Autodesk Inventor part; units mm, degrees
(part 8 of 8)
  line L3438 (-10.9335, 45.6499) -> (-10.7357, 45.6499) construction
  line L3439 (-10.7357, 45.6499) -> (-10.6212, 45.7817) construction
  spline S1087 degree 2 poles (-10.6212, 45.7817) (-10.5171, 45.8997) (-10.5171, 46.0697) knots 0 0 0 1 1 1
  line L3440 (-10.6212, 45.7817) -> (-10.5171, 45.8997) construction
  line L3441 (-10.5171, 45.8997) -> (-10.5171, 46.0697) construction
  spline S1088 degree 2 poles (-10.5171, 46.0697) (-10.5171, 46.4409) (-10.878, 46.4791) knots 0 0 0 1 1 1
  line L3442 (-10.5171, 46.0697) -> (-10.5171, 46.4409) construction
  line L3443 (-10.5171, 46.4409) -> (-10.878, 46.4791) construction
  line L3444 (-10.878, 46.4791) -> (-11.1382, 46.4791)
  circle A70 centre (18.7074, -0.5093) radius 2.3333
  circle A71 centre (12.3767, 19.6182) radius 2.3333
  circle A72 centre (-8.6685, 63.1738) radius 2.3333
  circle A73 centre (7.9982, 63.1738) radius 2.3333
  circle A74 centre (3.1182, 73.7406) radius 2.3333
  circle A75 centre (-12.2369, -33.319) radius 2.3333
  circle A76 centre (17.5807, -32.3391) radius 2.3333
  circle A77 centre (0.1742, -74.3888) radius 1.8001
  circle A78 centre (7.1838, -70.3418) radius 1.8001
  circle A79 centre (-6.8355, -78.4359) radius 1.8
  circle A80 centre (-4.5413, -27.5841) radius 2.3333
  circle A81 centre (11.7025, 73.7406) radius 2.3333
  circle A82 centre (7.9982, 57.3405) radius 2.3333
  circle A83 centre (-8.6685, 57.3405) radius 2.3333
  circle A84 centre (18.7074, -8.8426) radius 2.3333
  circle A85 centre (-3.7926, -8.8426) radius 2.3333
  circle A86 centre (5.7517, 15.6786) radius 2.3333
  circle A87 centre (-17.0018, 57.3405) radius 2.3333
  circle A88 centre (-0.3351, 57.3405) radius 2.3333
  circle A89 centre (17.9982, 57.3405) radius 2.3333
  circle A90 centre (-12.2369, -27.5841) radius 2.3333
  circle A91 centre (17.5807, -25.9665) radius 2.3333
  circle A92 centre (-6.8355, -70.3418) radius 1.8
  circle A93 centre (7.1838, -78.4359) radius 1.8001
  circle A94 centre (0.1742, -82.4829) radius 1.8001
  circle A95 centre (0.1742, -66.2948) radius 1.8001
  circle A96 centre (-4.5413, -33.319) radius 2.3333
  circle A97 centre (19.747, 73.7406) radius 2.3333
  circle A98 centre (17.9982, 63.1738) radius 2.3333
  circle A99 centre (-0.3351, 63.1738) radius 2.3333
  circle A100 centre (-17.0018, 63.1738) radius 2.3333
  circle A101 centre (0.2865, 19.6182) radius 2.3333
  circle A102 centre (-3.7926, -0.5093) radius 2.3333
  circle A103 centre (25.8333, -89.5833) radius 1.25
  circle A104 centre (-25.8333, -89.5833) radius 1.25
  circle A105 centre (25.8333, 89.5833) radius 1.25
  circle A106 centre (-25.8333, 89.5833) radius 1.25
  point P0 (0, 0)
  dimension "d0" = 3.6
  dimension "d1" = 3.6
  constraints: 1802 end point, 136 point on circle, 107 centre point, 3267 other
  measures "d0" diameter of A92
  measures "d1" diameter of A79
extrude "Выдавливание1" add sketch "Эскиз1" along normal blind 2 contours A68 S25 L514 S17 | S17 L514 S25 A68 S29 S28 L543 L3131 S968 S967 L399 L397 S966 S965 L3122 | L3122 S965 S966 L397 A68 | L543 S28 S29 A68 | A68 L399 S967 S968 L3131
sketch "Эскиз2" plane through (0.1742, -74.3888, 2) normal (0, 0, 1) x (1, 0, 0)
  circle A0 centre (0, 0) radius 1.8001 projected
  circle A1 centre (7.0097, 4.047) radius 1.8001 projected
  circle A2 centre (-7.0097, -4.047) radius 1.8 projected
  circle A3 centre (-7.0097, 4.047) radius 1.8 projected
  circle A4 centre (7.0097, -4.047) radius 1.8001 projected
  circle A5 centre (0, -8.0941) radius 1.8001 projected
  circle A6 centre (0, 8.0941) radius 1.8001 projected
  circle A7 centre (0, 0) radius 11.3681 projected
  line L0 (-3.147, 9.3371) -> (-3.147, 14.337)
  line L1 (-3.147, 14.337) -> (7.8973, 14.337)
  line L2 (7.8973, 14.337) -> (7.8973, 6.7447)
  line L3 (7.8973, 6.7447) -> (6.4258, 6.4788)
  line L4 (6.4258, 6.4788) -> (1.6002, 10.7812)
  line L5 (1.6002, 10.7812) -> (0.2827, 10.7812)
  line L6 (0.2827, 10.7812) -> (-3.147, 9.3371)
  point P0 (-0.1742, 74.3888)
  point P1 (-3.147, 10.9238)
  point P2 (6.84, 6.5537)
  point P3 (7.8973, 8.1772)
  constraints: 14 end point, 2 perpendicular, 1 parallel, 1 vertical
extrude "Выдавливание3" add sketch "Эскиз2" against normal blind 10 contours A7 L0 L1 L2
